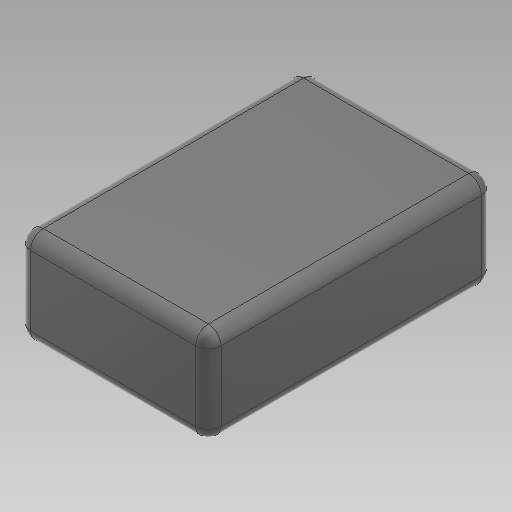
# Autodesk Inventor part: RBPI
Saved by Autodesk Inventor 2020 (Build 240168000, 168)
## iProperties
Created: 2022-08-27
Part Number: RBPI
Material: Acetal Resin, Black
Document SubType Name: Modeling
Designer: Umair
Density: 1.425 g/cm^3
Appearance: Smooth - Black
Author: Umair
Autodesk Inventor part; units mm, degrees
ref_plane "YZ Plane" through (0, 0, 0) normal (1, 0, 0) x (0, 1, 0)
ref_plane "XZ Plane" through (0, 0, 0) normal (0, 1, 0) x (-1, 0, 0)
ref_plane "XY Plane" through (0, 0, 0) normal (0, 0, 1) x (1, 0, 0)
sketch "Sketch1" plane through (0, 0, 0) normal (0, 1, 0) x (-1, 0, 0)
  line L0 (30, 45) -> (-30, 45)
  line L1 (-30, 45) -> (-30, -45)
  line L2 (-30, -45) -> (30, -45)
  line L3 (30, -45) -> (30, 45)
  line L4 (30, 45) -> (-30, -45) construction
  line L5 (-30, 45) -> (30, -45) construction
  point P0 (0, 0)
  dimension "d0" = 60
  dimension "d1" = 90
  constraints: 12 end point, 2 midpoint, 2 parallel, 1 horizontal, 1 perpendicular
  measures "d0" distance of L2.end L1.end
  measures "d1" distance of L1.end L0.end
extrude "Extrusion1" add sketch "Sketch1" along normal blind 30
fillet "Fillet1" radius 4 12 edges at (0, 30, -45) (0, 0, -45) (-30, 15, -45) (-30, 30, 0) (-30, 0, 0) (-30, 15, 45) (0, 30, 45) (0, 0, 45) (30, 15, 45) (30, 30, 0) (30, 15, -45) (30, 0, 0)
body "Solid1"
